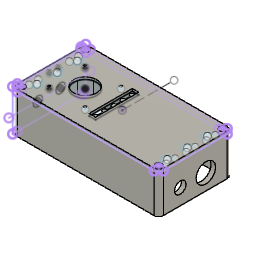
ROLEC 4x8 Joystick Module v1 (Autodesk Fusion 360 design; units mm, degrees)
Autodesk Fusion 360 part; units mm, degrees
sketch "Sketch1" plane through (0, 0, 0) normal (0, 1, 0) x (1, 0, 0)
  line L0 (95.25, 50.8) -> (-95.25, 50.8)
  line L1 (-101.6, 44.45) -> (-101.6, -44.45)
  line L2 (-95.25, -50.8) -> (95.25, -50.8)
  line L3 (101.6, -44.45) -> (101.6, 44.45)
  line L4 (101.6, 50.8) -> (-101.6, -50.8) construction
  line L5 (-101.6, 50.8) -> (101.6, -50.8) construction
  arc A0 (-95.25, 50.8) -> (-101.6, 44.45) centre (-95.25, 44.45) ccw
  arc A1 (-101.6, -44.45) -> (-95.25, -50.8) centre (-95.25, -44.45) ccw
  arc A2 (95.25, -50.8) -> (101.6, -44.45) centre (95.25, -44.45) ccw
  arc A3 (101.6, 44.45) -> (95.25, 50.8) centre (95.25, 44.45) ccw
  circle A4 centre (-95.25, 44.45) radius 4.7625
  circle A5 centre (-95.25, -44.45) radius 4.7625
  circle A6 centre (95.25, 44.45) radius 4.7625
  circle A7 centre (95.25, -44.45) radius 4.7625
  line L6 (-95.25, -44.45) -> (95.25, -44.45)
  line L7 (90.4875, 44.45) -> (-95.25, 44.45)
  line L8 (-95.25, 44.45) -> (-95.25, -44.45)
  arc A8 (-95.25, 33.3375) -> (-84.1375, 44.45) centre (-95.25, 44.45) ccw
  arc A9 (-84.1375, -44.45) -> (-95.25, -33.3375) centre (-95.25, -44.45) ccw
  arc A10 (95.25, -33.3375) -> (84.1375, -44.45) centre (95.25, -44.45) ccw
  arc A11 (84.1375, 44.45) -> (95.25, 33.3375) centre (95.25, 44.45) ccw
  line L9 (95.25, -44.45) -> (95.25, 33.3375)
  line L10 (95.25, 39.6875) -> (95.25, 44.45)
  dimension "d1" = 203.2
  dimension "d2" = 101.6
  dimension "d3" = 6.35
  dimension "d4" = 6.35
  dimension "d5" = 6.35
  dimension "d6" = 6.35
  dimension "d7" = 9.525
  dimension "d8" = 9.525
  dimension "d9" = 9.525
  dimension "d10" = 9.525
  dimension "d11" = 22.225
  dimension "d12" = 22.225
  dimension "d13" = 22.225
  dimension "d14" = 22.225
  constraint horizontal L0
  constraint perpendicular L0 L1
  constraint parallel L0 L2
  constraint parallel L1 L3
  constraint coincident L4 origin
  constraint coincident L5 origin
  constraint coincident L5.start L1
  constraint coincident L5.start L0
  constraint tangent L1 A0
  constraint tangent L0 A0
  constraint coincident L4.end L2
  constraint coincident L4.end L1
  constraint tangent L2 A1
  constraint tangent L1 A1
  constraint coincident L5.end L2
  constraint coincident L5.end L3
  constraint tangent L2 A2
  constraint tangent L3 A2
  constraint coincident L4.start L0
  constraint coincident L4.start L3
  constraint tangent L0 A3
  constraint tangent L3 A3
  constraint concentric A0 A4
  constraint concentric A1 A5
  constraint concentric A3 A6
  constraint concentric A2 A7
  constraint concentric A0 A8
  constraint concentric A6 A11
  constraint concentric A2 A10
  constraint concentric A1 A9
  constraint coincident L8 A8.start
  constraint coincident L7 A8.end
  constraint coincident L8 A9.end
  constraint coincident L6 A9.start
  constraint coincident A10.start L9
  constraint coincident L6 A10.end
  constraint coincident L7 A11.start
  constraint coincident A6 L10.start
  constraint collinear L9 L10
  constraint coincident A6 L7.start
  measures "d1" distance of L4.end L5.end
  measures "d2" distance of L5.start L4.end
  measures "d3" radius of A0
  measures "d4" radius of A1
  measures "d5" radius of A2
  measures "d6" radius of A3
  measures "d7" diameter of A4
  measures "d8" diameter of A5
  measures "d9" diameter of A6
  measures "d10" diameter of A7
  measures "d11" diameter of A8
  measures "d12" diameter of A11
  measures "d13" diameter of A10
  measures "d14" diameter of A9
extrude "Extrude1" add sketch "Sketch1" against normal blind 23.8125 contours L0 L1 L2 L3 A0 A1 A2 A3 | A4 L7 L8 A8 | A5 L6 L8 A9 | A7 L6 A10 L9 makes body 1 in component "Joystick Module lid"
sketch "Sketch1 (2)" plane through (0, -23.8125, 0) normal (0, -1, 0) x (1, 0, 0) in component "Joystick Module lid"
  circle A0 centre (95.25, -44.45) radius 4.7625
  circle A1 centre (-95.25, -44.45) radius 4.7625
  circle A2 centre (-95.25, 44.45) radius 4.7625
  line L0 (84.1375, -44.45) -> (-84.1375, -44.45)
  arc A3 (-84.1375, -44.45) -> (-95.25, -33.3375) centre (-95.25, -44.45) ccw
  line L1 (-95.25, -33.3375) -> (-95.25, 33.3375)
  arc A4 (-95.25, 33.3375) -> (-84.1375, 44.45) centre (-95.25, 44.45) ccw
  line L2 (-84.1375, 44.45) -> (84.1375, 44.45)
  arc A5 (84.1375, 44.45) -> (95.25, 33.3375) centre (95.25, 44.45) ccw
  line L3 (95.25, 33.3375) -> (95.25, -33.3375)
  arc A6 (95.25, -33.3375) -> (84.1375, -44.45) centre (95.25, -44.45) ccw
  circle A7 centre (95.25, 44.45) radius 4.7625
  arc A8 (95.25, -50.8) -> (101.6, -44.45) centre (95.25, -44.45) ccw
  line L4 (101.6, -44.45) -> (101.6, 44.45)
  arc A9 (101.6, 44.45) -> (95.25, 50.8) centre (95.25, 44.45) ccw
  line L5 (95.25, 50.8) -> (-95.25, 50.8)
  arc A10 (-95.25, 50.8) -> (-101.6, 44.45) centre (-95.25, 44.45) ccw
  line L6 (-101.6, 44.45) -> (-101.6, -44.45)
  arc A11 (-101.6, -44.45) -> (-95.25, -50.8) centre (-95.25, -44.45) ccw
  line L7 (-95.25, -50.8) -> (95.25, -50.8)
  line L8 (-101.6, -44.45) -> (-101.6, 44.45)
  line L9 (-95.25, 50.8) -> (95.25, 50.8)
  arc A12 (-95.25, 50.8) -> (-101.6, 44.45) centre (-95.25, 44.45) ccw
  line L10 (95.25, -50.8) -> (-95.25, -50.8)
  arc A13 (-101.6, -44.45) -> (-95.25, -50.8) centre (-95.25, -44.45) ccw
  arc A14 (95.25, -50.8) -> (101.6, -44.45) centre (95.25, -44.45) ccw
  line L11 (101.6, 44.45) -> (101.6, -44.45)
  arc A15 (101.6, 44.45) -> (95.25, 50.8) centre (95.25, 44.45) ccw
  circle A16 centre (95.25, 44.45) radius 4.7625
  circle A17 centre (-95.25, 44.45) radius 4.7625
  circle A18 centre (-95.25, -44.45) radius 4.7625
  circle A19 centre (95.25, -44.45) radius 4.7625
extrude "Extrude2" add sketch "Sketch1 (2)" along normal blind 3.175 contours L0 A3 L1 A4 L2 A5 L3 A6 | A8 L4 A9 L5 A10 L6 A11 L7 L8 L9 A12 L10 A13 A14 L11 A15 bodies 1 in component "Joystick Module lid"
sketch "bottom sketch" plane through (0, 0, 0) normal (0, 1, 0) x (1, 0, 0) in component "Joystick Module base"
  arc A0 (84.1375, 44.45) -> (95.25, 33.3375) centre (95.25, 44.45) ccw
  line L0 (84.1375, 44.45) -> (-84.1375, 44.45)
  arc A1 (-95.25, 33.3375) -> (-84.1375, 44.45) centre (-95.25, 44.45) ccw
  line L1 (-95.25, 33.3375) -> (-95.25, -33.3375)
  arc A2 (-84.1375, -44.45) -> (-95.25, -33.3375) centre (-95.25, -44.45) ccw
  line L2 (-84.1375, -44.45) -> (84.1375, -44.45)
  arc A3 (95.25, -33.3375) -> (84.1375, -44.45) centre (95.25, -44.45) ccw
  line L3 (95.25, -33.3375) -> (95.25, 33.3375)
  line L4 (101.6, -44.45) -> (101.6, 44.45)
  arc A4 (101.6, 44.45) -> (95.25, 50.8) centre (95.25, 44.45) ccw
  line L5 (95.25, 50.8) -> (-95.25, 50.8)
  arc A5 (95.25, -50.8) -> (101.6, -44.45) centre (95.25, -44.45) ccw
  line L6 (-95.25, -50.8) -> (95.25, -50.8)
  arc A6 (-95.25, 50.8) -> (-101.6, 44.45) centre (-95.25, 44.45) ccw
  line L7 (-101.6, 44.45) -> (-101.6, -44.45)
  arc A7 (-101.6, -44.45) -> (-95.25, -50.8) centre (-95.25, -44.45) ccw
  circle A8 centre (-95.25, -44.45) radius 4.7625
  circle A9 centre (-95.25, 44.45) radius 4.7625
  circle A10 centre (95.25, 44.45) radius 4.7625
  circle A11 centre (95.25, -44.45) radius 4.7625
extrude "Extrude1'" add sketch "bottom sketch" along normal blind 53.975 separate body makes body 2 in component "Joystick Module base"
sketch "top sketch" plane through (0, 53.975, 0) normal (0, 1, 0) x (-1, 0, 0) in component "Joystick Module base"
  circle A0 centre (95.25, 44.45) radius 4.7625
  circle A1 centre (95.25, -44.45) radius 4.7625
  circle A2 centre (-95.25, -44.45) radius 4.7625
  circle A3 centre (-95.25, 44.45) radius 4.7625
  line L0 (-84.1375, 44.45) -> (84.1375, 44.45)
  arc A4 (84.1375, 44.45) -> (95.25, 33.3375) centre (95.25, 44.45) ccw
  line L1 (95.25, 33.3375) -> (95.25, -33.3375)
  arc A5 (95.25, -33.3375) -> (84.1375, -44.45) centre (95.25, -44.45) ccw
  line L2 (84.1375, -44.45) -> (-84.1375, -44.45)
  arc A6 (-84.1375, -44.45) -> (-95.25, -33.3375) centre (-95.25, -44.45) ccw
  line L3 (-95.25, -33.3375) -> (-95.25, 33.3375)
  arc A7 (-95.25, 33.3375) -> (-84.1375, 44.45) centre (-95.25, 44.45) ccw
  arc A8 (101.6, 44.45) -> (95.25, 50.8) centre (95.25, 44.45) ccw
  line L4 (95.25, 50.8) -> (-95.25, 50.8)
  arc A9 (-95.25, 50.8) -> (-101.6, 44.45) centre (-95.25, 44.45) ccw
  line L5 (-101.6, 44.45) -> (-101.6, -44.45)
  arc A10 (-101.6, -44.45) -> (-95.25, -50.8) centre (-95.25, -44.45) ccw
  line L6 (-95.25, -50.8) -> (95.25, -50.8)
  arc A11 (95.25, -50.8) -> (101.6, -44.45) centre (95.25, -44.45) ccw
  line L7 (101.6, -44.45) -> (101.6, 44.45)
  circle A12 centre (95.25, -44.45) radius 4.7625
  line L8 (-95.25, -50.8) -> (95.25, -50.8)
  arc A13 (95.25, -50.8) -> (101.6, -44.45) centre (95.25, -44.45) ccw
  arc A14 (101.6, 44.45) -> (95.25, 50.8) centre (95.25, 44.45) ccw
  line L9 (95.25, 50.8) -> (-95.25, 50.8)
  arc A15 (-101.6, -44.45) -> (-95.25, -50.8) centre (-95.25, -44.45) ccw
  line L10 (-101.6, 44.45) -> (-101.6, -44.45)
  arc A16 (-95.25, 50.8) -> (-101.6, 44.45) centre (-95.25, 44.45) ccw
  circle A17 centre (-95.25, 44.45) radius 4.7625
  circle A18 centre (-95.25, -44.45) radius 4.7625
  circle A19 centre (51.6, 0) radius 16
  line L11 (101.6, -44.45) -> (101.6, 44.45)
  line L12 (101.6, -44.45) -> (101.6, 44.45)
  circle A20 centre (76.6, -25) radius 1.5
  circle A21 centre (76.6, 25) radius 1.5
  circle A22 centre (26.6, -25) radius 1.5
  circle A23 centre (26.6, 25) radius 1.5
  line L13 (16, -30) -> (7, -30)
  line L14 (7, -30) -> (7, 30)
  line L15 (7, 30) -> (16, 30)
  line L16 (16, 30) -> (16, -30)
  line L17 (-90.4875, -44.45) -> (95.25, -44.45)
  line L18 (90.6, -6.25) -> (95.25, -6.25)
  line L19 (90.6, 6.25) -> (95.25, 6.25)
  arc A24 (90.6, 6.25) -> (90.6, -6.25) centre (90.6, 0) ccw
  circle A25 centre (90.6, 0) radius 2
  line L20 (90.5837, 21.7502) -> (95.25, 21.7059)
  arc A26 (90.7026, 34.2497) -> (90.5837, 21.7502) centre (90.6431, 28) ccw
  line L21 (90.7026, 34.2497) -> (95.25, 34.2064)
  circle A27 centre (90.6431, 28) radius 2
  line L22 (90.6, -34.25) -> (95.25, -34.25)
  arc A28 (90.6, -21.75) -> (90.6, -34.25) centre (90.6, -28) ccw
  line L23 (90.6, -21.75) -> (95.25, -21.75)
  circle A29 centre (90.6, -28) radius 2
  line L24 (0, 0) -> (0, -72.1921) construction
  arc A30 (-90.6, -34.25) -> (-90.6, -21.75) centre (-90.6, -28) ccw
  line L25 (-90.6, -34.25) -> (-95.25, -34.25)
  line L26 (-90.6, -21.75) -> (-95.25, -21.75)
  circle A31 centre (-90.6, -28) radius 2
  line L27 (-90.6, -6.25) -> (-95.25, -6.25)
  arc A32 (-90.6, -6.25) -> (-90.6, 6.25) centre (-90.6, 0) ccw
  circle A33 centre (-90.6, 0) radius 2
  line L28 (-90.6, 6.25) -> (-95.25, 6.25)
  line L29 (-90.5837, 21.7502) -> (-95.25, 21.7059)
  arc A34 (-90.5837, 21.7502) -> (-90.7026, 34.2497) centre (-90.6431, 28) ccw
  circle A35 centre (-90.6431, 28) radius 2
  line L30 (-90.7026, 34.2497) -> (-95.25, 34.2064)
  dimension "d22" = 32
  dimension "d23" = 50
  dimension "d24" = 3
  dimension "d25" = 25
  dimension "d26" = 25
  dimension "d27" = 3
  dimension "d28" = 25
  dimension "d29" = 25
  dimension "d30" = 3
  dimension "d31" = 3
  dimension "d32" = 9
  dimension "d33" = 60
  dimension "d35" = 50.8
  dimension "d36" = 50.8
  dimension "d37" = 20.8
  dimension "d38" = 20.8
  dimension "d39" = 108.6
  dimension "d40" = 203.2
  dimension "d65" = 12.5
  dimension "d66" = 11
  dimension "d67" = 4
  dimension "d68" = 12.5
  dimension "d69" = 4
  dimension "d70" = 28
  dimension "d71" = 12.5
  dimension "d72" = 4
  dimension "d73" = 28
  dimension "d76" = 50
  dimension "d77" = 50
  constraint horizontal L13
  constraint vertical L14
  constraint horizontal L15
  constraint vertical L16
  constraint coincident L1 L18.end
  constraint tangent L18 A24
  constraint perpendicular L1 L18
  constraint coincident L1 L19.end
  constraint tangent L19 A24
  constraint perpendicular L1 L19
  constraint concentric A24 A25
  constraint tangent L20 A26
  constraint tangent A26 L21
  constraint concentric A26 A27
  constraint tangent L22 A28
  constraint tangent A28 L23
  constraint concentric A28 A29
  constraint coincident L24.start origin
  constraint perpendicular L8 L24
  constraint symmetric L18.start L24 L27.start
  constraint symmetric L18.end L24 L27.end
  constraint symmetric L19.start L24 A32.end
  constraint symmetric L19.end L24 L28.end
  constraint symmetric A24 L24 A32
  constraint symmetric A25 L24 A33
  constraint symmetric L20.end L24 L29.end
  constraint symmetric L20.start L24 L29.start
  constraint symmetric A26.start L24 A34.end
  constraint symmetric L21.end L24 L30.end
  constraint symmetric A26 L24 A34
  constraint symmetric A27 L24 A35
  constraint symmetric L22.end L24 L25.end
  constraint symmetric L22.start L24 A30.start
  constraint symmetric A28.start L24 A30.end
  constraint symmetric L23.end L24 L26.end
  constraint symmetric A28 L24 A30
  constraint symmetric A29 L24 A31
  measures "d22" diameter of A19
  measures "d23" distance of A19.centre L11
  measures "d24" diameter of A20
  measures "d25" vertical distance of A19.centre A20.centre
  measures "d26" horizontal distance of A19.centre A20.centre
  measures "d27" diameter of A21
  measures "d28" horizontal distance of A19.centre A21.centre
  measures "d29" vertical distance of A19.centre A21.centre
  measures "d30" diameter of A22
  measures "d31" diameter of A23
  measures "d32" distance of L13.start L13.end
  measures "d33" distance of L13.end L14.end
  measures "d35" distance of L8 A19.centre
  measures "d36" distance of L9 A19.centre
  measures "d37" distance of L9 L15
  measures "d38" distance of L6 L13.end
  measures "d39" distance of L10 L14
  measures "d40" distance of L10 L11
  measures "d65" diameter of A24
  measures "d66" distance of L7 A24.centre
  measures "d67" diameter of A25
  measures "d68" diameter of A26
  measures "d69" diameter of A27
  measures "d70" distance of A24.centre A26.centre
  measures "d71" diameter of A28
  measures "d72" diameter of A29
  measures "d73" distance of A24.centre A28.centre
  measures "d76" distance of A20.centre A22.centre
  measures "d77" distance of A21.centre A23.centre
extrude "Extrude2'" add sketch "top sketch" along normal blind 3.175 contours L0 A4 L1 A5 L2 A6 L3 A7 L17 L18 L19 A24 L20 A26 L21 L22 A28 L23 A30 L25 L26 L27 A32 L28 L29 A34 L30 | L3 A7 L29 A34 L30 | A4 L1 L20 A26 L21 | L3 L27 A32 L28 | L1 L18 L19 A24 | A6 L3 A30 L25 L26 | L1 A5 L22 A28 L23 | A8 L4 A9 L5 A10 L6 A11 L7 L8 A13 A14 L9 A15 L10 A16 L11 L12 | A25 | A27 | A29 | A31 | A33 | A35 bodies 2 in component "Joystick Module base"
sketch "Sketch1 (3)" plane through (0, 57.15, 0) normal (0, 1, 0) x (-1, 0, 0) in component "top overlay"
  circle A0 centre (26.6, 25) radius 1.5
  circle A1 centre (76.6, -25) radius 1.5
  circle A2 centre (51.6, 0) radius 16
  circle A3 centre (76.6, 25) radius 1.5
  circle A4 centre (-95.25, -44.45) radius 4.7625
  circle A5 centre (95.25, 44.45) radius 4.7625
  circle A6 centre (95.25, -44.45) radius 4.7625
  circle A7 centre (-95.25, 44.45) radius 4.7625
  line L0 (7, 30) -> (16, 30)
  line L1 (16, 30) -> (16, -30)
  line L2 (16, -30) -> (7, -30)
  line L3 (7, -30) -> (7, 30)
  circle A8 centre (26.6, -25) radius 1.5
  line L4 (101.6, -44.45) -> (101.6, 44.45)
  arc A9 (101.6, 44.45) -> (95.25, 50.8) centre (95.25, 44.45) ccw
  line L5 (95.25, 50.8) -> (-95.25, 50.8)
  arc A10 (-95.25, 50.8) -> (-101.6, 44.45) centre (-95.25, 44.45) ccw
  line L6 (-101.6, 44.45) -> (-101.6, -44.45)
  arc A11 (-101.6, -44.45) -> (-95.25, -50.8) centre (-95.25, -44.45) ccw
  line L7 (-95.25, -50.8) -> (95.25, -50.8)
  arc A12 (95.25, -50.8) -> (101.6, -44.45) centre (95.25, -44.45) ccw
  circle A13 centre (51.6, 0) radius 16
  line L8 (11.5, -73.7068) -> (11.5, -68.5116)
  line L9 (11.5, -68.5116) -> (11.5, 73.0574) construction
  line L10 (-101.6, 44.45) -> (-101.6, -44.45) construction
  line L11 (7, -30) -> (7, 30) construction
  line L12 (16, 30) -> (16, -30) construction
  line L13 (0, 0) -> (24.4686, 0) construction
  line L14 (8, -3.5) -> (15, -3.5)
  line L15 (15, -3.5) -> (15, 3.5)
  line L16 (15, 3.5) -> (8, 3.5)
  line L17 (8, 3.5) -> (8, -3.5)
  line L18 (8, -3.5) -> (15, 3.5) construction
  line L19 (15, -3.5) -> (8, 3.5) construction
  line L20 (15, -16.2) -> (15, -9.2)
  line L21 (8, -16.2) -> (15, -16.2)
  line L22 (8, -9.2) -> (8, -16.2)
  line L23 (15, -9.2) -> (8, -9.2)
  line L24 (15, 16.2) -> (8, 16.2)
  line L25 (15, 9.2) -> (15, 16.2)
  line L26 (8, 9.2) -> (15, 9.2)
  line L27 (8, 16.2) -> (8, 9.2)
  line L28 (8, 28.9) -> (8, 21.9)
  line L29 (8, 21.9) -> (15, 21.9)
  line L30 (15, 21.9) -> (15, 28.9)
  line L31 (15, 28.9) -> (8, 28.9)
  line L32 (15, -21.9) -> (8, -21.9)
  line L33 (8, -21.9) -> (8, -28.9)
  line L34 (15, -28.9) -> (15, -21.9)
  line L35 (8, -28.9) -> (15, -28.9)
  line L36 (99.6, -44.45) -> (99.6, 44.45)
  arc A14 (99.6, 44.45) -> (95.25, 48.8) centre (95.25, 44.45) ccw
  line L37 (95.25, 48.8) -> (-95.25, 48.8)
  arc A15 (-95.25, 48.8) -> (-99.6, 44.45) centre (-95.25, 44.45) ccw
  line L38 (-99.6, 44.45) -> (-99.6, -44.45)
  arc A16 (-99.6, -44.45) -> (-95.25, -48.8) centre (-95.25, -44.45) ccw
  line L39 (-95.25, -48.8) -> (95.25, -48.8)
  arc A17 (95.25, -48.8) -> (99.6, -44.45) centre (95.25, -44.45) ccw
  line L40 (1.9647, 30.565) -> (1.8348, 19.842) construction
  line L41 (1.8348, 19.842) -> (3.9774, 19.816) construction
  line L42 (3.9774, 19.816) -> (4.1073, 30.539) construction
  line L43 (4.1073, 30.539) -> (1.9647, 30.565) construction
  line L44 (1.9647, 17.865) -> (1.8348, 7.142) construction
  line L45 (1.8348, 7.142) -> (3.9774, 7.116) construction
  line L46 (3.9774, 7.116) -> (4.1073, 17.839) construction
  line L47 (4.1073, 17.839) -> (1.9647, 17.865) construction
  line L48 (1.9647, 5.165) -> (1.8348, -5.558) construction
  line L49 (1.8348, -5.558) -> (3.9774, -5.584) construction
  line L50 (3.9774, -5.584) -> (4.1073, 5.139) construction
  line L51 (4.1073, 5.139) -> (1.9647, 5.165) construction
  line L52 (1.9647, -7.535) -> (1.8348, -18.258) construction
  line L53 (1.8348, -18.258) -> (3.9774, -18.284) construction
  line L54 (3.9774, -18.284) -> (4.1073, -7.561) construction
  line L55 (4.1073, -7.561) -> (1.9647, -7.535) construction
  line L56 (1.9647, -20.235) -> (1.8348, -30.958) construction
  line L57 (1.8348, -30.958) -> (3.9774, -30.984) construction
  line L58 (3.9774, -30.984) -> (4.1073, -20.261) construction
  line L59 (4.1073, -20.261) -> (1.9647, -20.235) construction
  point P0 (26.6, -25)
  point P1 (76.6, -25)
  point P2 (76.6, 25)
  point P3 (26.6, 25)
  point P4 (11.5, 0)
  dimension "d45" = 9
  dimension "d46" = 4.5
  dimension "d47" = 7
  dimension "d48" = 7
  dimension "d49" = 7
  dimension "d50" = 7
  dimension "d51" = 7
  dimension "d52" = 7
  dimension "d53" = 7
  dimension "d54" = 7
  dimension "d55" = 7
  dimension "d56" = 7
  dimension "d57" = -2
  dimension "d60" = 2
  dimension "d61" = 2
  dimension "d62" = 2
  dimension "d63" = 2
  dimension "d64" = 2
  constraint vertical L8
  constraint parallel L1 L9
  constraint coincident L13.start origin
  constraint perpendicular L12 L13
  constraint horizontal L14
  constraint perpendicular L14 L15
  constraint parallel L14 L16
  constraint parallel L15 L17
  constraint coincident L18 P4
  constraint coincident L19 P4
  constraint coincident L13 P4
  constraint coincident L9 P4
  constraint horizontal L21
  constraint perpendicular L20 L21
  constraint parallel L21 L23
  constraint parallel L20 L22
  constraint horizontal L26
  constraint perpendicular L25 L26
  constraint parallel L24 L26
  constraint parallel L25 L27
  constraint horizontal L29
  constraint perpendicular L29 L30
  constraint parallel L29 L31
  constraint parallel L28 L30
  constraint horizontal L35
  constraint perpendicular L34 L35
  constraint parallel L32 L35
  constraint parallel L33 L34
  measures "d45" distance of L11 L12
  measures "d46" distance of L9 L2.end
  measures "d47" distance of L15.end L16.end
  measures "d48" distance of L14.end L15.end
  measures "d49" distance of L20.end L22.start
  measures "d50" distance of L20.start L20.end
  measures "d51" distance of L24.start L24.end
  measures "d52" distance of L25.start L24.start
  measures "d53" distance of L28.start L30.end
  measures "d54" distance of L29.end L30.end
  measures "d55" distance of L32.start L32.end
  measures "d56" distance of L32.start L34.start
extrude "Extrude1''" add sketch "Sketch1 (3)" along normal blind 1 separate body contours A4 L38 A16 L39 | A4 A5 A6 A7 L36 L37 L38 L39 | A7 L37 A15 L38 | A6 L36 L39 A17 | A5 L36 A14 L37 | L0 L1 L2 L3 picked at (-95.5027, -44.8575) picked at (-95.5027, 44.8575) picked at (95.5775, -44.7775) picked at (95.5775, 44.7775) makes body 3 in component "top overlay"
extrude "Extrude3" add sketch "top sketch" against normal blind 6 contours L3 A7 L29 A34 L30 | A4 L1 L20 A26 L21 | L3 L27 A32 L28 | L1 L18 L19 A24 | A6 L3 A30 L25 L26 | L1 A5 L22 A28 L23 bodies 2 in component "Joystick Module base"
sketch "back face" plane through (101.6, 0, 0) normal (1, 0, 0) x (0, 0, -1) in component "Joystick Module base"
  line L0 (-44.45, 0) -> (44.45, 0)
  line L1 (44.45, 0) -> (44.45, 57.15)
  line L2 (44.45, 57.15) -> (-44.45, 57.15)
  line L3 (-44.45, 57.15) -> (-44.45, 0)
  line L4 (-50.8, 0) -> (-50.8, 57.15)
  line L5 (-44.45, 0) -> (44.45, 0)
  line L6 (50.8, 0) -> (44.45, 0)
  line L7 (50.8, 0) -> (50.8, 57.15)
  line L8 (-44.45, 57.15) -> (44.45, 57.15)
  line L9 (-44.45, 57.15) -> (-50.8, 57.15)
  line L10 (50.8, 57.15) -> (44.45, 57.15)
  line L11 (-56.1109, 22) -> (57.2916, 22) construction
  circle A0 centre (14.8, 22) radius 13.5
  circle A1 centre (-20.8, 22) radius 8
  circle A2 centre (14.8, 22) radius 17 construction
  circle A3 centre (-20.8, 22) radius 11 construction
  circle A4 centre (14.8, 22) radius 18.5 construction
  point P0 (0, 53.975)
  dimension "d78" = 22
  dimension "d79" = 27
  dimension "d80" = 16
  dimension "d81" = 34
  dimension "d84" = 22
  dimension "d85" = 37
  dimension "d88" = 36
  dimension "d89" = 30
  constraint perpendicular L7 L11
  constraint coincident L11 A0.centre
  constraint coincident L11 A1.centre
  constraint concentric A0 A2
  constraint concentric A1 A3
  constraint concentric A2 A4
  measures "d78" distance of L5 L11
  measures "d79" diameter of A0
  measures "d80" diameter of A1
  measures "d81" diameter of A2
  measures "d84" diameter of A3
  measures "d85" diameter of A4
  measures "d88" distance of L7 A0.centre
  measures "d89" distance of L4 A1.centre
extrude "Extrude4" cut sketch "back face" against normal blind 10 contours A0 | A1 bodies 2 in component "Joystick Module base"
sketch "Sketch4" plane through (-101.6, 0, 0) normal (-1, 0, 0) x (0, 0, 1) in component "Joystick Module base"
  line L0 (-44.45, 0) -> (44.45, 0)
  line L1 (44.45, 0) -> (44.45, 57.15)
  line L2 (44.45, 57.15) -> (-44.45, 57.15)
  line L3 (-44.45, 57.15) -> (-44.45, 0)
  line L4 (-50.8, 0) -> (-50.8, 57.15)
  line L5 (44.45, 0) -> (-44.45, 0)
  line L6 (44.45, 57.15) -> (-44.45, 57.15)
  line L7 (50.8, 0) -> (50.8, 57.15)
  line L8 (50.8, 0) -> (44.45, 0)
  line L9 (-50.8, 0) -> (-44.45, 0)
  line L10 (56.1109, 22) -> (-57.2916, 22)
  line L11 (-50.8, 57.15) -> (-44.45, 57.15)
  line L12 (44.45, 57.15) -> (50.8, 57.15)
  circle A0 centre (15.8, 22) radius 6.35
  circle A1 centre (-15.8, 22) radius 6.35
  dimension "d90" = 12.7
  dimension "d91" = 12.7
  dimension "d92" = 35
  dimension "d93" = 35
  constraint coincident L10 A0.centre
  constraint coincident L10 A1.centre
  measures "d90" diameter of A0
  measures "d91" diameter of A1
  measures "d92" distance of L4 A1.centre
  measures "d93" distance of L7 A0.centre
extrude "Extrude5" cut sketch "Sketch4" against normal blind 10 contours L10 A1 | L10 A1 | L10 A0 | L10 A0 bodies 2 in component "Joystick Module base"
sketch "Sketch1 (4)" plane through (0, 47.975, 0) normal (0, -1, 0) x (1, 0, 0) in component "Mk VI PCB profile"
  circle A0 centre (90.6431, 28) radius 2
  arc A1 (90.7026, 34.2497) -> (90.5837, 21.7502) centre (90.6431, 28) ccw
  line L0 (90.5837, 21.7502) -> (95.25, 21.7059)
  line L1 (95.25, 21.7059) -> (95.25, 33.3375)
  arc A2 (90.8439, 34.2483) -> (95.25, 33.3375) centre (95.25, 44.45) ccw
  line L2 (90.8439, 34.2483) -> (90.7026, 34.2497)
  circle A3 centre (-76.6, 25) radius 1.5
  circle A4 centre (-76.6, -25) radius 1.5
  circle A5 centre (-51.6, 0) radius 16
  circle A6 centre (-26.6, -25) radius 1.5
  circle A7 centre (-26.6, 25) radius 1.5
  line L3 (-16, 30) -> (-7, 30)
  line L4 (-7, 30) -> (-7, -30)
  line L5 (-7, -30) -> (-16, -30)
  line L6 (-16, -30) -> (-16, 30)
  line L7 (95.25, 21.7059) -> (90.5837, 21.7502)
  arc A8 (90.7026, 34.2497) -> (90.5837, 21.7502) centre (90.6431, 28) ccw
  line L8 (90.7026, 34.2497) -> (90.8439, 34.2483)
  arc A9 (84.1375, 44.45) -> (90.8439, 34.2483) centre (95.25, 44.45) ccw
  line L9 (84.1375, 44.45) -> (-84.1375, 44.45)
  arc A10 (-90.8439, 34.2483) -> (-84.1375, 44.45) centre (-95.25, 44.45) ccw
  line L10 (-90.8439, 34.2483) -> (-90.7026, 34.2497)
  arc A11 (-90.5837, 21.7502) -> (-90.7026, 34.2497) centre (-90.6431, 28) ccw
  line L11 (-90.5837, 21.7502) -> (-95.25, 21.7059)
  line L12 (-95.25, 21.7059) -> (-95.25, 6.25)
  line L13 (-95.25, 6.25) -> (-90.6, 6.25)
  arc A12 (-90.6, -6.25) -> (-90.6, 6.25) centre (-90.6, 0) ccw
  line L14 (-90.6, -6.25) -> (-95.25, -6.25)
  line L15 (-95.25, -6.25) -> (-95.25, -21.75)
  line L16 (-95.25, -21.75) -> (-90.6, -21.75)
  arc A13 (-90.6, -34.25) -> (-90.6, -21.75) centre (-90.6, -28) ccw
  line L17 (-90.6, -34.25) -> (-90.8401, -34.25)
  arc A14 (-84.1375, -44.45) -> (-90.8401, -34.25) centre (-95.25, -44.45) ccw
  line L18 (-84.1375, -44.45) -> (84.1375, -44.45)
  arc A15 (90.8401, -34.25) -> (84.1375, -44.45) centre (95.25, -44.45) ccw
  line L19 (90.8401, -34.25) -> (90.6, -34.25)
  arc A16 (90.6, -21.75) -> (90.6, -34.25) centre (90.6, -28) ccw
  line L20 (90.6, -21.75) -> (95.25, -21.75)
  line L21 (95.25, -21.75) -> (95.25, -6.25)
  line L22 (95.25, -6.25) -> (90.6, -6.25)
  arc A17 (90.6, 6.25) -> (90.6, -6.25) centre (90.6, 0) ccw
  line L23 (90.6, 6.25) -> (95.25, 6.25)
  line L24 (95.25, 6.25) -> (95.25, 21.7059)
  line L25 (-7, -30) -> (-7, 30)
  line L26 (-16, 30) -> (-16, -30)
  line L27 (-16, -30) -> (-7, -30)
  line L28 (-7, 30) -> (-16, 30)
  circle A18 centre (-51.6, 0) radius 16
  circle A19 centre (90.6431, 28) radius 2.5
  circle A20 centre (90.6, -28) radius 2.5
  line L29 (-17.3569, 44) -> (82.1434, 44)
  line L30 (94.6431, 31.5) -> (94.6431, -31.5)
  line L31 (82.1431, -44) -> (-17.3569, -44)
  line L32 (-17.3569, -44) -> (-17.3569, 44)
  arc A21 (94.6431, -31.5) -> (82.1431, -44) centre (94.6431, -44) ccw
  arc A22 (82.1434, 44) -> (94.6431, 31.5) centre (94.6434, 44) ccw
  line L33 (50.1051, 41.7153) -> (78.1051, 41.7153)
  line L34 (78.1051, 41.7153) -> (78.1051, 28.7153)
  line L35 (78.1051, 28.7153) -> (50.1051, 28.7153)
  line L36 (50.1051, 28.7153) -> (50.1051, 41.7153)
  line L37 (-3.6868, 20.4275) -> (58.3132, 20.4275)
  line L38 (58.3132, 20.4275) -> (58.3132, -12.5725)
  line L39 (58.3132, -12.5725) -> (-3.6868, -12.5725)
  line L40 (-3.6868, -12.5725) -> (-3.6868, 20.4275)
  line L41 (0.2045, 34.1616) -> (43.2045, 34.1616)
  line L42 (43.2045, 34.1616) -> (43.2045, 21.1616)
  line L43 (43.2045, 21.1616) -> (0.2045, 21.1616)
  line L44 (0.2045, 21.1616) -> (0.2045, 34.1616)
  line L45 (63.6103, -8.4141) -> (73.6103, -8.4141)
  line L46 (73.6103, -8.4141) -> (73.6103, -36.4141)
  line L47 (73.6103, -36.4141) -> (63.6103, -36.4141)
  line L48 (63.6103, -36.4141) -> (63.6103, -8.4141)
  line L49 (21.2635, -31.7621) -> (40.4912, -31.7621)
  line L50 (40.4912, -31.7621) -> (40.4912, -39.3159)
  line L51 (40.4912, -39.3159) -> (21.2635, -39.3159)
  line L52 (21.2635, -39.3159) -> (21.2635, -31.7621)
  circle A23 centre (35.5165, -22.2255) radius 6.5
  circle A24 centre (-11.5, 0) radius 3
  circle A25 centre (-11.5, 12.7) radius 3
  circle A26 centre (-11.5, 25.4) radius 3
  circle A27 centre (-11.5, -12.7) radius 3
  circle A28 centre (-11.5, -25.4) radius 3
  line L53 (-11.5, -68.5116) -> (-11.5, 73.0574)
  point P0 (90.6431, 28)
  point P1 (90.6, 0)
  point P2 (90.6, -28)
  point P3 (-51.6, 0)
  point P4 (-11.5, 0)
  dimension "d96" = 5
  dimension "d97" = 5
  dimension "d99" = 88
  dimension "d100" = 4
  dimension "d101" = 16
  dimension "d103" = 12.5
  dimension "d104" = 12.5
  dimension "d105" = 12.5
  dimension "d106" = 12.5
  dimension "d107" = 112
  dimension "d108" = 28
  dimension "d109" = 13
  dimension "d110" = 62
  dimension "d111" = 33
  dimension "d112" = 43
  dimension "d113" = 13
  dimension "d114" = 10
  dimension "d115" = 28
  dimension "d116" = 13
  dimension "d117" = 6
  dimension "d118" = 6
  dimension "d119" = 6
  dimension "d120" = 6
  dimension "d121" = 6
  dimension "d122" = 12.7
  dimension "d123" = 12.7
  dimension "d124" = 12.7
  dimension "d125" = 12.7
  constraint coincident P0 A0.centre
  constraint coincident P2 A16.centre
  constraint horizontal L29
  constraint vertical L30
  constraint horizontal L31
  constraint vertical L32
  constraint horizontal L33
  constraint vertical L34
  constraint horizontal L35
  constraint vertical L36
  constraint horizontal L37
  constraint vertical L38
  constraint horizontal L39
  constraint vertical L40
  constraint horizontal L41
  constraint vertical L42
  constraint horizontal L43
  constraint vertical L44
  constraint horizontal L45
  constraint vertical L46
  constraint horizontal L47
  constraint vertical L48
  constraint horizontal L49
  constraint vertical L50
  constraint horizontal L51
  constraint vertical L52
  constraint coincident P4 A24.centre
  measures "d96" diameter of A19
  measures "d97" diameter of A20
  measures "d99" distance of L29.start L31.end
  measures "d100" distance of P0 L30
  measures "d101" distance of P0 L29
  measures "d103" radius of A21
  measures "d104" distance of A22.centre L30.start
  measures "d105" horizontal distance of L29.end A22.centre
  measures "d106" distance of A21.centre L31.start
  measures "d107" distance of L30 L32
  measures "d108" distance of L33.start L33.end
  measures "d109" distance of L33.start L35.end
  measures "d110" distance of L37.start L37.end
  measures "d111" distance of L37.start L39.end
  measures "d112" distance of L41.start L41.end
  measures "d113" distance of L41.start L43.end
  measures "d114" distance of L45.start L45.end
  measures "d115" distance of L45.start L47.end
  measures "d116" diameter of A23
  measures "d117" diameter of A24
  measures "d118" diameter of A25
  measures "d119" diameter of A26
  measures "d120" diameter of A27
  measures "d121" diameter of A28
  measures "d122" distance of P4 A27.centre
  measures "d123" distance of A27.centre A28.centre
  measures "d124" distance of P4 A25.centre
  measures "d125" distance of A25.centre A26.centre
extrude "Extrude1'''" add sketch "Sketch1 (4)" along normal blind 2 separate body contours A1 L0 L7 A8 L30 A22 | A1 L0 L3 L4 L5 L7 A8 A16 L20 L22 A17 L23 L25 L27 L28 L29 L30 L31 A21 A22 L53 | L3 L5 L6 L26 L27 L28 L29 L31 L32 L53 | L22 A17 L23 L30 | L3 L5 L6 L26 L27 L28 A24 A25 A26 A27 A28 L53 | L3 L4 L5 L25 L27 L28 A24 A25 A26 A27 A28 L53 | A16 L20 L30 A21 makes body 4 in component "Mk VI PCB profile"
extrude "Extrude2''" add sketch "Sketch1 (4)" along normal blind 15 contours L41 L42 L43 L44 bodies 4 in component "Mk VI PCB profile"
extrude "Extrude3'" add sketch "Sketch1 (4)" along normal blind 26 contours L33 L34 L35 L36 bodies 4 in component "Mk VI PCB profile"
extrude "Extrude4'" add sketch "Sketch1 (4)" along normal blind 14 contours L37 L38 L39 L40 bodies 4 in component "Mk VI PCB profile"
extrude "Extrude5'" add sketch "Sketch1 (4)" along normal blind 13 contours L45 L46 L47 L48 bodies 4 in component "Mk VI PCB profile"
extrude "Extrude6" add sketch "Sketch1 (4)" along normal blind 7 contours A23 bodies 4 in component "Mk VI PCB profile"
extrude "Extrude7" add sketch "Sketch1 (4)" along normal blind 7 contours L49 L50 L51 L52 bodies 4 in component "Mk VI PCB profile"
extrude "Extrude8" add sketch "Sketch1 (4)" along normal blind -6 and the other way blind -2 contours A26 L53 | A26 L53 | A25 L53 | A25 L53 | A28 L53 | A28 L53 | A24 L53 | A24 L53 | A27 L53 | A27 L53 bodies 4 in component "Mk VI PCB profile"
sketch "Sketch3" plane through (0, 33.975, 0) normal (0, -1, 0) x (1, 0, 0) in component "Mk VI PCB profile"
  line L0 (-3.6868, -12.5725) -> (58.3132, -12.5725)
  line L1 (58.3132, -12.5725) -> (58.3132, 20.4275)
  line L2 (58.3132, 20.4275) -> (-3.6868, 20.4275)
  line L3 (-3.6868, 20.4275) -> (-3.6868, -12.5725)
  circle A0 centre (10.547, 27.7873) radius 5.5
  circle A1 centre (32.547, 27.7873) radius 5.5
  line L4 (51.9042, 10.3442) -> (57.9042, 10.3442)
  line L5 (57.9042, 10.3442) -> (57.9042, 0.3442)
  line L6 (57.9042, 0.3442) -> (51.9042, 0.3442)
  line L7 (51.9042, 0.3442) -> (51.9042, 10.3442)
  line L8 (51.9042, -0.8113) -> (57.9042, -0.8113)
  line L9 (57.9042, -0.8113) -> (57.9042, -10.8113)
  line L10 (57.9042, -10.8113) -> (51.9042, -10.8113)
  line L11 (51.9042, -10.8113) -> (51.9042, -0.8113)
  circle A2 centre (45.3132, -6.5725) radius 5
  circle A3 centre (33.3132, -6.5725) radius 5
  line L12 (-2.1002, 9.3266) -> (1.9773, 9.3266)
  line L13 (1.9773, 9.3266) -> (1.9773, -0.7651)
  line L14 (1.9773, -0.7651) -> (-2.1002, -0.7651)
  line L15 (-2.1002, -0.7651) -> (-2.1002, 9.3266)
  dimension "d144" = 11
  dimension "d145" = 11
  dimension "d146" = 22
  dimension "d147" = 6
  dimension "d148" = 10
  dimension "d149" = 6
  dimension "d150" = 10
  dimension "d151" = 10
  dimension "d152" = 10
  dimension "d153" = 12
  dimension "d154" = 13
  dimension "d155" = 6
  constraint horizontal L4
  constraint vertical L5
  constraint horizontal L6
  constraint vertical L7
  constraint horizontal L8
  constraint vertical L9
  constraint horizontal L10
  constraint vertical L11
  constraint collinear L7 L11
  constraint horizontal L12
  constraint vertical L13
  constraint horizontal L14
  constraint vertical L15
  measures "d144" diameter of A0
  measures "d145" diameter of A1
  measures "d146" distance of A0.centre A1.centre
  measures "d147" distance of L4.start L4.end
  measures "d148" distance of L4.start L6.end
  measures "d149" distance of L8.start L8.end
  measures "d150" distance of L8.start L10.end
  measures "d151" diameter of A2
  measures "d152" diameter of A3
  measures "d153" distance of A2.centre A3.centre
  measures "d154" distance of L1 A2.centre
  measures "d155" distance of L0 A2.centre
extrude "Extrude9" add sketch "Sketch3" along normal blind 10 contours L4 L5 L6 L7 | L8 L9 L10 L11 | A2 | A3 bodies 4 in component "Mk VI PCB profile"
extrude "Extrude10" add sketch "Sketch3" along normal blind 6 contours L12 L13 L14 L15 bodies 4 in component "Mk VI PCB profile"
extrude "Extrude11" add sketch "Sketch3" along normal blind 8 contours A0 | A1 bodies 4 in component "Mk VI PCB profile"
sketch "Sketch4 (2)" plane through (0, 25.975, 0) normal (0, -1, 0) x (1, 0, 0) in component "Mk VI PCB profile"
  circle A0 centre (32.547, 27.7873) radius 5.5
  circle A1 centre (32.547, 27.7873) radius 2
  circle A2 centre (10.547, 27.7873) radius 2
  point P0 (10.547, 27.7873)
  dimension "d162" = 4
  dimension "d163" = 4
  constraint concentric A0 A1
  constraint coincident P0 A2.centre
  measures "d162" diameter of A1
  measures "d163" diameter of A2
extrude "Extrude12" add sketch "Sketch4 (2)" along normal blind 7 contours A1 | A2 bodies 4 in component "Mk VI PCB profile"
component "Joystick Module lid" placed x (1, 0, 0) y (0, 1, 0) z (0, 0, 1) at (0, 0, 0)
component "Joystick Module base" placed x (1, 0, 0) y (0, 1, 0) z (0, 0, 1) at (0, 0, 0)
component "top overlay" placed x (1, 0, 0) y (0, 1, 0) z (0, 0, 1) at (0, 0, 0)
component "Mk VI PCB profile" placed x (1, 0, 0) y (0, 1, 0) z (0, 0, 1) at (0, 0, 0)
equation "d11 = 0.375 in + 0.50 in"
equation "d12 = d11"
equation "d13 = d11"
equation "d14 = d11"
equation "d27 = d24"
equation "d30 = d24"
equation "d31 = d24"
equation "d38 = d35 - d33 / 2"
equation "d39 = 110 mm - d32 / 2 + 3.1 mm"
equation "d73 = d70"
equation "d77 = d76"
equation "d93 = d92"
equation "d105 = d104"
named bodies: "Rolex 4x8 lid"
